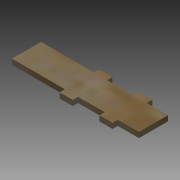
# Autodesk Inventor part: hlid
Saved by Autodesk Inventor 2015 (Build 190159000, 159)
## iProperties
Created: 2015-10-06
Part Number: hlid
Material: Generic
Document SubType Name: Modeling
Designer: Haukur
Density: 1 g/cm^3
Appearance: Plywood - Weathered
Author: Haukur
Autodesk Inventor part; units mm, degrees
ref_plane "YZ Plane" through (0, 0, 0) normal (1, 0, 0) x (0, 1, 0)
ref_plane "XZ Plane" through (0, 0, 0) normal (0, 1, 0) x (-1, 0, 0)
ref_plane "XY Plane" through (0, 0, 0) normal (0, 0, 1) x (1, 0, 0)
sketch "Sketch1" plane through (0, 0, 0) normal (0, 0, 1) x (1, 0, 0)
  line L0 (0, 4) -> (0, 26)
  line L1 (0, 26) -> (40, 26)
  line L2 (40, 26) -> (40, 30)
  line L3 (40, 30) -> (50, 30)
  line L4 (50, 30) -> (50, 26)
  line L5 (50, 26) -> (70, 26)
  line L6 (70, 26) -> (70, 30)
  line L7 (70, 30) -> (80, 30)
  line L8 (80, 30) -> (80, 26)
  line L9 (80, 26) -> (96, 26)
  line L10 (96, 26) -> (96, 4)
  line L11 (96, 4) -> (80, 4)
  line L12 (80, 4) -> (80, 0)
  line L13 (80, 0) -> (70, 0)
  line L14 (70, 0) -> (70, 4)
  line L15 (70, 4) -> (50, 4)
  line L16 (50, 4) -> (50, 0)
  line L17 (50, 0) -> (40, 0)
  line L18 (40, 4) -> (0, 4)
  line L19 (40, 0) -> (40, 4)
  point P0 (0, 0)
  dimension "d0" = 22
  dimension "d1" = 40
  dimension "d2" = 4
  dimension "d3" = 10
  dimension "d4" = 20
  dimension "d5" = 10
  dimension "d6" = 16
  constraints: 40 end point, 19 point on line, 11 perpendicular, 1 vertical
  measures "d0" distance of L0.start L0.end
  measures "d1" distance of L0.end L1.end
  measures "d2" distance of L1.end L2.end
  measures "d3" distance of L2.end L3.end
  measures "d4" distance of L4.end L5.end
  measures "d5" distance of L6.end L7.end
  measures "d6" distance of L8.end L9.end
extrude "Extrusion1" add sketch "Sketch1" along normal blind 4
body "Solid1"
